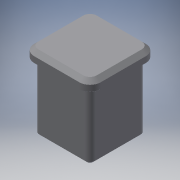
# Autodesk Inventor part: nút nhựa bit hộp thép 25x25
Saved by Autodesk Inventor 2016 (Build 200138000, 138)
## iProperties
Created: 2018-11-05
Part Number: nút nhựa bit hộp thép 25x25
Material: Generic
Document SubType Name: Modeling
Designer: hovm
Density: 1 g/cm^3
Appearance: Default
Author: hovm
Autodesk Inventor part; units mm, degrees
ref_plane "YZ Plane" through (0, 0, 0) normal (1, 0, 0) x (0, 1, 0)
ref_plane "XZ Plane" through (0, 0, 0) normal (0, 1, 0) x (-1, 0, 0)
ref_plane "XY Plane" through (0, 0, 0) normal (0, 0, 1) x (1, 0, 0)
sketch "Sketch1" plane through (0, 0, 0) normal (0, 0, 1) x (1, 0, 0)
  line L0 (8.5, 10.5) -> (-8.5, 10.5) projected
  line L1 (8.5, 10.5) -> (-8.5, 10.5) projected
  arc A0 (10.5, 8.5) -> (8.5, 10.5) centre (8.5, 8.5) ccw projected
  line L2 (10.5, -8.5) -> (10.5, 8.5) projected
  arc A1 (8.5, -10.5) -> (10.5, -8.5) centre (8.5, -8.5) ccw projected
  line L3 (-8.5, -10.5) -> (8.5, -10.5) projected
  arc A2 (-10.5, -8.5) -> (-8.5, -10.5) centre (-8.5, -8.5) ccw projected
  line L4 (-10.5, 8.5) -> (-10.5, -8.5) projected
  arc A3 (-8.5, 10.5) -> (-10.5, 8.5) centre (-8.5, 8.5) ccw projected
  line L5 (-12.5, -8.5) -> (-12.5, 8.5) projected
  arc A4 (-12.5, -8.5) -> (-8.5, -12.5) centre (-8.5, -8.5) ccw projected
  line L6 (8.5, -12.5) -> (-8.5, -12.5) projected
  arc A5 (8.5, -12.5) -> (12.5, -8.5) centre (8.5, -8.5) ccw projected
  line L7 (12.5, 8.5) -> (12.5, -8.5) projected
  arc A6 (12.5, 8.5) -> (8.5, 12.5) centre (8.5, 8.5) ccw projected
  line L8 (-8.5, 12.5) -> (8.5, 12.5) projected
  arc A7 (-8.5, 12.5) -> (-12.5, 8.5) centre (-8.5, 8.5) ccw projected
  point P0 (0, 0)
extrude "Extrusion1" add sketch "Sketch1" against normal blind 25 contours A0 L2 A1 L3 A2 L4 A3 L0
sketch "Sketch2" plane through (0, 0, 0) normal (0, 0, 1) x (1, 0, 0)
  line L0 (8.5, 10.5) -> (-8.5, 10.5) projected
  arc A0 (10.5, 8.5) -> (8.5, 10.5) centre (8.5, 8.5) ccw projected
  line L1 (10.5, -8.5) -> (10.5, 8.5) projected
  arc A1 (8.5, -10.5) -> (10.5, -8.5) centre (8.5, -8.5) ccw projected
  line L2 (-8.5, -10.5) -> (8.5, -10.5) projected
  arc A2 (-10.5, -8.5) -> (-8.5, -10.5) centre (-8.5, -8.5) ccw projected
  line L3 (-10.5, 8.5) -> (-10.5, -8.5) projected
  arc A3 (-8.5, 10.5) -> (-10.5, 8.5) centre (-8.5, 8.5) ccw projected
  line L4 (-12.5, -8.5) -> (-12.5, 8.5) projected
  arc A4 (-12.5, -8.5) -> (-8.5, -12.5) centre (-8.5, -8.5) ccw projected
  line L5 (8.5, -12.5) -> (-8.5, -12.5) projected
  arc A5 (8.5, -12.5) -> (12.5, -8.5) centre (8.5, -8.5) ccw projected
  line L6 (12.5, 8.5) -> (12.5, -8.5) projected
  arc A6 (12.5, 8.5) -> (8.5, 12.5) centre (8.5, 8.5) ccw projected
  line L7 (-8.5, 12.5) -> (8.5, 12.5) projected
  arc A7 (-8.5, 12.5) -> (-12.5, 8.5) centre (-8.5, 8.5) ccw projected
  point P0 (0, 0)
extrude "Extrusion2" add sketch "Sketch2" along normal blind 4 contours A0 L1 A1 L2 A2 L3 A3 L0 | L4 A7 L7 A6 L6 A5 L5 A4
chamfer "Chamfer1" distance 1 angle 45 8 edges at (0, 10.5, -25) (9.9142, 9.9142, -25) (10.5, 0, -25) (9.9142, -9.9142, -25) (0, -10.5, -25) (-9.9142, -9.9142, -25) (-10.5, 0, -25) (-9.9142, 9.9142, -25)
chamfer "Chamfer2" distance 1.5 angle 45 8 edges at (0, 12.5, 4) (-11.3284, 11.3284, 4) (-12.5, 0, 4) (-11.3284, -11.3284, 4) (0, -12.5, 4) (11.3284, -11.3284, 4) (12.5, 0, 4) (11.3284, 11.3284, 4)
chamfer "Chamfer3" distance 0.3 angle 45 8 edges at (0, 12.5, 0) (11.3284, 11.3284, 0) (12.5, 0, 0) (11.3284, -11.3284, 0) (0, -12.5, 0) (-11.3284, -11.3284, 0) (-12.5, 0, 0) (-11.3284, 11.3284, 0)
body "Solid1"
